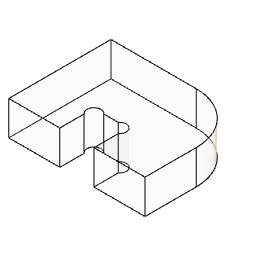
rotation sensor plate v1 (Autodesk Fusion 360 archive; units mm, degrees)
design "rotation sensor plate" references "Global Parameters"
Autodesk Fusion 360 part; units mm, degrees
derive "Derived from Global Parameters v5" from "Global Parameters v5"
sketch "Sketch1" plane through (0, 0, 0) normal (0, 0, 1) x (1, 0, 0)
  line L0 (0, 0) -> (40, 0)
  line L1 (40, 0) -> (40, 20)
  line L2 (40, 20) -> (0, 20)
  line L3 (0, 20) -> (0, 0)
  line L4 (0, 0) -> (15, 0)
  line L5 (15, 0) -> (15, -10)
  line L6 (15, -10) -> (0, -10)
  line L7 (0, -10) -> (0, 0)
  line L8 (40, 0) -> (25, 0)
  line L9 (25, 0) -> (25, -10)
  line L10 (25, -10) -> (40, -10)
  line L11 (40, -10) -> (40, 0)
  line L12 (15, 0) -> (16.2728, -1.2728) construction
  line L13 (15, 0) -> (16.8, 0) construction
  line L14 (25, 0) -> (23.7272, -1.2728) construction
  line L15 (25, 0) -> (23.2, 0) construction
  dimension "d1" = 20
  dimension "d2" = 40
  dimension "d5" = 15
  dimension "d6" = 10
  dimension "d7" = 15
  dimension "d8" = 10
  dimension "d13" = 45
  dimension "d14" = 1.8
  dimension "d15" = 45
  dimension "d16" = 1.8
  constraint horizontal L0
  constraint vertical L1
  constraint horizontal L2
  constraint vertical L3
  constraint coincident L0.start L3.end
  constraint horizontal L4
  constraint vertical L5
  constraint horizontal L6
  constraint vertical L7
  constraint horizontal L8
  constraint vertical L9
  constraint horizontal L10
  constraint vertical L11
  constraint horizontal L13
  constraint horizontal L15
  measures "d1" distance of L0.start L2.end
  measures "d2" distance of L1.end L2.end
  measures "d5" distance of L0.start L4.end
  measures "d6" distance of L0.start L6.end
  measures "d7" distance of L0.end L8.end
  measures "d8" distance of L0.end L10.end
  measures "d13" angle of L12 L13
  measures "d14" distance of L4.end L12.end
  measures "d15" angle of L14 L15
  measures "d16" distance of L8.end L14.end
extrude "Extrude1" add sketch "Sketch1" along normal blind 10
fillet "Fillet1" radius 15 1 edges at (40, 20, 5)
sketch "Sketch2" plane through (0, 0, 0) normal (-1, 0, 0) x (0, -1, 0)
  line L0 (-20, 0) -> (10, 0)
  line L1 (10, 0) -> (10, 10)
  line L2 (10, 10) -> (-20, 10)
  line L3 (-20, 10) -> (-20, 0)
  line L4 (-20, 5) -> (10, 5)
  constraint midpoint L3 L4.start
  constraint midpoint L1 L4.end
hole "Hole1" at (23.7272, -1.2728, 0) at (16.2728, -1.2728, 0) direction (0, 0, 1) diameter 4.1 end through all
equation "pmma_thickness_Ref = 10 mm" comment "The thickness of the Perspex (Poly Methyl Meth Acrylaat) plate"
equation "rotate_motor_Ref = 117 deg"
equation "d6 = pmma_thickness_Ref"
equation "d8 = pmma_thickness_Ref"
equation "d9 = pmma_thickness_Ref"
